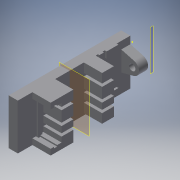
# Autodesk Inventor part: Assembly-jig-base
Saved by Autodesk Inventor 2018 (Build 220112000, 112)
## iProperties
Created: 2017-11-08
Part Number: Assembly-jig-base
Material: Generic
Document SubType Name: Modeling
Designer: xl0
Density: 1 g/cm^3
Appearance: Default
Author: xl0
Autodesk Inventor part; units mm, degrees
ref_plane "YZ Plane" through (0, 0, 0) normal (1, 0, 0) x (0, 1, 0)
ref_plane "XZ Plane" through (0, 0, 0) normal (0, 1, 0) x (-1, 0, 0)
ref_plane "XY Plane" through (0, 0, 0) normal (0, 0, 1) x (1, 0, 0)
ref_plane "Work Plane3" through (-2, 0, -40) normal (-1, 0, 0) x (0, 0, 1)
sketch "Sketch3" plane through (-2, 0, -8) normal (-1, 0, 0) x (0, -1, 0)
  line L0 (59.7526, 13.1) -> (72.7526, 13.1)
  line L1 (72.7526, 13.1) -> (72.7526, 3.1)
  line L2 (72.7526, 3.1) -> (59.7526, 3.1)
  line L3 (59.7526, 3.1) -> (59.7526, 13.1)
  line L4 (104.2526, 13.1) -> (117.2526, 13.1)
  line L5 (117.2526, 13.1) -> (117.2526, 3.1)
  line L6 (117.2526, 3.1) -> (104.2526, 3.1)
  line L7 (104.2526, 3.1) -> (104.2526, 13.1)
  line L8 (59.7526, -25.1) -> (72.7526, -25.1)
  line L9 (72.7526, -25.1) -> (72.7526, -35.1)
  line L10 (72.7526, -35.1) -> (59.7526, -35.1)
  line L11 (59.7526, -35.1) -> (59.7526, -25.1)
  line L12 (104.2526, -25.1) -> (117.2526, -25.1)
  line L13 (117.2526, -25.1) -> (117.2526, -35.1)
  line L14 (117.2526, -35.1) -> (104.2526, -35.1)
  line L15 (104.2526, -35.1) -> (104.2526, -25.1)
  line L16 (41.7526, -32) -> (41.7526, 8) projected
  line L17 (125.2526, 8) -> (125.2526, -32) projected
  line L18 (63.2526, 0) -> (63.2526, 3) projected
  line L19 (67.7526, 0) -> (67.7526, 3) projected
  line L20 (99.2526, 0) -> (99.2526, 3) projected
  line L21 (103.7526, 0) -> (103.7526, 3) projected
  line L22 (44.7526, 3) -> (122.2526, 3) projected
  line L23 (122.2526, -25) -> (44.7526, -25) projected
  line L24 (74.7526, -0.1) -> (87.7526, -0.1)
  line L25 (87.7526, -0.1) -> (87.7526, -11.9)
  line L26 (87.7526, -11.9) -> (74.7526, -11.9)
  line L27 (74.7526, -11.9) -> (74.7526, -0.1)
  line L28 (59.7526, -15.1) -> (72.7526, -15.1)
  line L29 (72.7526, -15.1) -> (72.7526, -21.9)
  line L30 (72.7526, -21.9) -> (59.7526, -21.9)
  line L31 (59.7526, -21.9) -> (59.7526, -15.1)
  line L32 (104.2526, -0.1) -> (117.2526, -0.1)
  line L33 (117.2526, -0.1) -> (117.2526, -11.9)
  line L34 (117.2526, -11.9) -> (104.2526, -11.9)
  line L35 (104.2526, -11.9) -> (104.2526, -0.1)
  line L36 (104.2526, -15.1) -> (117.2526, -15.1)
  line L37 (117.2526, -15.1) -> (117.2526, -21.9)
  line L38 (117.2526, -21.9) -> (104.2526, -21.9)
  line L39 (104.2526, -21.9) -> (104.2526, -15.1)
  line L40 (44.7526, 0) -> (122.2526, 0) projected
  line L41 (44.7526, -12) -> (122.2526, -12) projected
  line L42 (44.7526, -15) -> (122.2526, -15) projected
  line L43 (44.7526, -22) -> (122.2526, -22) projected
  line L44 (122.2526, 8) -> (122.2526, -32) projected
  line L45 (44.7526, -32) -> (44.7526, 8) projected
  line L46 (125.2526, 8) -> (122.2526, 8) projected
  line L47 (125.2526, -32) -> (122.2526, -32) projected
  dimension "d7" = 10
  dimension "d9" = 0.1
  dimension "d10" = 0.1
  dimension "d11" = 0.1
  dimension "d12" = 0.1
  dimension "d13" = 0.1
  dimension "d34" = 5
  dimension "d36" = 13
  dimension "d48" = 0.1
  dimension "d49" = 15
  dimension "d67" = 15
  constraints: 64 end point, 16 parallel, 14 collinear, 8 horizontal, 8 perpendicular, 4 equal length, 3 point on line
  measures "d7" distance of L0.end L1.end
  measures "d9" distance between parallel lines of L23 L8
  measures "d10" distance between parallel lines of L26 L41
  measures "d11" distance between parallel lines of L40 L24
  measures "d12" distance between parallel lines of L42 L28
  measures "d13" distance between parallel lines of L43 L30
  measures "d34" distance between parallel lines of L37 L44
  measures "d36" distance of L9.end L10.end
  measures "d48" distance between parallel lines of L22 L2
  measures "d49" distance between parallel lines of L45 L31
  measures "d67" distance between parallel lines of L27 L31
extrude "Extrusion2" add sketch "Sketch3" against normal blind 20 contours L0 L1 L2 L3 | L4 L5 L6 L7 | L8 L9 L10 L11 | L12 L13 L14 L15 | L24 L25 L26 L27 | L28 L29 L30 L31 | L32 L33 L34 L35 | L36 L37 L38 L39
sketch "Sketch10" plane through (-2, 0, -8) normal (-1, 0, 0) x (0, 0, 1)
  line L0 (13.1, -117.2526) -> (13.1, -129.2526)
  line L1 (13.1, -129.2526) -> (6.7, -129.2526)
  line L2 (6.7, -129.2526) -> (6.7, -125.4526)
  line L3 (6.7, -125.4526) -> (8.2, -125.4526)
  line L4 (6.7, -117.2526) -> (13.1, -117.2526)
  line L5 (8, -125.2526) -> (-32, -125.2526) projected
  line L6 (8, -125.2526) -> (8, -122.2526) projected
  line L7 (-32, -122.2526) -> (8, -122.2526) projected
  line L8 (-32, -125.2526) -> (-32, -122.2526) projected
  line L9 (13.1, -104.2526) -> (13.1, -117.2526) projected
  line L10 (-30.7, -129.2526) -> (-37.1, -129.2526)
  line L11 (-37.1, -129.2526) -> (-37.1, -104.2526)
  line L12 (-32.2, -125.4526) -> (-30.7, -125.4526)
  line L13 (-30.7, -125.4526) -> (-30.7, -129.2526)
  line L14 (-32.2, -125.4526) -> (-32.2, -122.0526)
  line L15 (-32.2, -122.0526) -> (-30.7, -122.0526)
  line L16 (-30.7, -122.0526) -> (-30.7, -117.2526)
  line L17 (8.2, -125.4526) -> (8.2, -122.0526)
  line L18 (8.2, -122.0526) -> (6.7, -122.0526)
  line L19 (6.7, -122.0526) -> (6.7, -117.2526)
  line L20 (13.1, -117.2526) -> (3.1, -117.2526) projected
  line L21 (-25.1, -104.2526) -> (-25.1, -117.2526) projected
  line L22 (-25.1, -117.2526) -> (-35.1, -117.2526) projected
  line L23 (-35.1, -117.2526) -> (-35.1, -104.2526) projected
  line L24 (-35.1, -104.2526) -> (-25.1, -104.2526) projected
  line L25 (-35.1, -117.2526) -> (-35.1, -104.2526) projected
  line L26 (-35.1, -104.2526) -> (-37.1, -104.2526)
  point P0 (8, 0)
  dimension "d50" = 0.2
  dimension "d54" = 12
  dimension "d58" = 0.2
  dimension "d59" = 0.2
  dimension "d60" = 1.5
  dimension "d61" = 0.2
  constraints: 32 end point, 9 collinear, 7 perpendicular, 3 horizontal, 3 parallel, 2 vertical, 1 point on line
  measures "d50" distance between parallel lines of L3 L5
  measures "d54" distance of L0.start L0.end
  measures "d58" distance between parallel lines of L17 L6
  measures "d59" distance between parallel lines of L18 L7
  measures "d60" distance of L17.end L18.end
  measures "d61" distance between parallel lines of L8 L14
extrude "Extrusion7" add sketch "Sketch10" against normal blind 20 contours L0 L1 L2 L3 L17 L18 L19 L4 | L10 L11 L26 L23 L22 L16 L15 L14 L12 L13
sketch "Sketch11" plane through (-2, 0, -8) normal (-1, 0, 0) x (0, 0, 1)
  line L0 (6.7, -122.0526) -> (6.7, -117.2526) projected
  line L1 (8.2, -122.0526) -> (6.7, -122.0526) projected
  line L2 (8.2, -125.4526) -> (8.2, -122.0526) projected
  line L3 (6.7, -125.4526) -> (8.2, -125.4526) projected
  line L4 (6.7, -129.2526) -> (6.7, -125.4526) projected
  line L5 (13.1, -129.2526) -> (6.7, -129.2526) projected
  line L6 (-37.1, -129.2526) -> (-30.7, -129.2526) projected
  line L7 (-30.7, -129.2526) -> (-30.7, -125.4526) projected
  line L8 (-30.7, -125.4526) -> (-32.2, -125.4526) projected
  line L9 (-32.2, -125.4526) -> (-32.2, -122.0526) projected
  line L10 (-32.2, -122.0526) -> (-30.7, -122.0526) projected
  line L11 (-30.7, -122.0526) -> (-30.7, -117.2526) projected
  line L12 (-37.1, -104.2526) -> (-37.1, -129.2526) projected
  line L13 (6.7, -122.0526) -> (6.7, -125.4526)
  line L14 (-30.7, -122.0526) -> (-32.2, -122.0526) projected
  line L15 (-30.7, -122.0526) -> (-30.7, -125.4526)
  line L16 (13.1, -36.7526) -> (6.1, -36.7526)
  line L17 (6.1, -36.7526) -> (6.1, -49.7526)
  line L18 (6.1, -49.7526) -> (13.1, -49.7526)
  line L19 (13.1, -49.7526) -> (13.1, -36.7526)
  line L20 (-28.1, -36.7526) -> (-35.1, -36.7526)
  line L21 (-35.1, -36.7526) -> (-35.1, -49.7526)
  line L22 (-35.1, -49.7526) -> (-28.1, -49.7526)
  line L23 (-28.1, -49.7526) -> (-28.1, -36.7526)
  line L24 (13.1, -59.7526) -> (13.1, -72.7526) projected
  line L25 (-35.1, -72.7526) -> (-35.1, -59.7526) projected
  line L26 (-11.9, -74.7526) -> (-0.1, -74.7526) projected
  line L27 (-32, -44.7526) -> (8, -44.7526)
  line L28 (-25.1, -104.2526) -> (-25.1, -117.2526) projected
  line L29 (-25.1, -117.2526) -> (-30.7, -117.2526) projected
  line L30 (13.1, -104.2526) -> (13.1, -129.2526) projected
  line L31 (3.1, -104.2526) -> (13.1, -104.2526) projected
  line L32 (3.1, -117.2526) -> (3.1, -104.2526) projected
  line L33 (6.7, -117.2526) -> (3.1, -117.2526) projected
  line L34 (-25.1, -104.2526) -> (-37.1, -104.2526) projected
  point P0 (8, 0)
  dimension "d64" = 7
  dimension "d65" = 5
  constraints: 22 end point, 5 collinear, 5 parallel, 3 horizontal, 3 perpendicular, 3 point on line, 2 other
  measures "d64" distance of L16.start L16.end
  measures "d65" distance between parallel lines of L22 L27
ref_plane "Work Plane5" through (0, -122.2526, -8) normal (-1, 0, 0) x (0, 0, 1)
extrude "Extrusion8" add sketch "Sketch11" against normal up to surface (2 mm away) contours L1 L2 L3 L13 | L12 L34 L28 L29 L11 L10 L9 L8 L7 L6 | L19 L18 L17 L16 | L23 L22 L21 L20
sketch "Sketch4" plane through (-2, 0, -8) normal (-1, 0, 0) x (0, 0, 1)
  line L0 (13.1, -21.7526) -> (-37.1, -21.7526)
  line L1 (-37.1, -21.7526) -> (-37.1, -130.2526)
  line L2 (-37.1, -130.2526) -> (13.1, -130.2526)
  line L3 (13.1, -130.2526) -> (13.1, -21.7526)
  line L4 (13.1, -59.7526) -> (13.1, -72.7526) projected
  line L5 (3.1, -59.7526) -> (13.1, -59.7526) projected
  line L6 (3.1, -72.7526) -> (3.1, -59.7526) projected
  line L7 (13.1, -72.7526) -> (3.1, -72.7526) projected
  line L8 (13.1, -104.2526) -> (13.1, -129.2526) projected
  line L9 (3.1, -104.2526) -> (13.1, -104.2526) projected
  line L10 (3.1, -117.2526) -> (3.1, -104.2526) projected
  line L11 (6.7, -117.2526) -> (3.1, -117.2526) projected
  line L12 (-25.1, -59.7526) -> (-25.1, -72.7526) projected
  line L13 (-35.1, -59.7526) -> (-25.1, -59.7526) projected
  line L14 (-35.1, -72.7526) -> (-35.1, -59.7526) projected
  line L15 (-25.1, -72.7526) -> (-35.1, -72.7526) projected
  line L16 (-25.1, -104.2526) -> (-25.1, -117.2526) projected
  line L17 (-25.1, -104.2526) -> (-37.1, -104.2526) projected
  line L18 (-25.1, -117.2526) -> (-30.7, -117.2526) projected
  line L19 (-32, -41.7526) -> (8, -41.7526) projected
  line L20 (8, -125.2526) -> (-32, -125.2526) projected
  line L21 (13.1, -59.7526) -> (13.1, -72.7526) projected
  line L22 (-35.1, -72.7526) -> (-35.1, -59.7526) projected
  line L23 (6.7, -129.2526) -> (6.7, -117.2526) projected
  line L24 (13.1, -129.2526) -> (6.7, -129.2526) projected
  line L25 (-37.1, -104.2526) -> (-37.1, -129.2526) projected
  line L26 (-37.1, -129.2526) -> (-30.7, -129.2526) projected
  line L27 (-30.7, -129.2526) -> (-30.7, -125.4526) projected
  line L28 (-30.7, -125.4526) -> (-32.2, -125.4526) projected
  line L29 (-32.2, -125.4526) -> (-32.2, -122.0526) projected
  line L30 (-32.2, -122.0526) -> (-30.7, -122.0526) projected
  line L31 (-30.7, -122.0526) -> (-30.7, -117.2526) projected
  line L32 (-37.1, -129.2526) -> (-37.1, -104.2526) projected
  point P0 (8, 0)
  dimension "d16" = 20
  dimension "d17" = 5
  constraints: 8 end point, 2 collinear, 2 parallel, 1 horizontal, 1 perpendicular
  measures "d16" distance between parallel lines of L0 L19
  measures "d17" distance between parallel lines of L2 L20
extrude "Extrusion3" add sketch "Sketch4" along normal blind 10 contours L3 L5 L6 L7 L9 L10 L11 L23 L24 L2 L1 L26 L27 L28 L29 L30 L31 L18 L16 L17 L0 | L3 L7 L6 L5 | L17 L16 L18 L31 L30 L29 L28 L27 L26 L1 | L3 L24 L23 L11 L10 L9 | L12 L15 L14 L13
sketch "Sketch5" plane through (-2, -21.7526, 5.1) normal (0, 1, 0) x (1, 0, 0)
  point P0 (2, 5.1)
sketch "Sketch6" plane through (-2, -21.7526, 5.1) normal (0, 1, 0) x (1, 0, 0)
  line L0 (26.75, 28.1) -> (18.75, 28.1) projected
  line L1 (18.75, 28.1) -> (18.75, 25.1) projected
  line L2 (26.75, 25.1) -> (18.75, 25.1) projected
  line L3 (26.75, 28.1) -> (26.75, 25.1) projected
  line L4 (26.75, 13.1) -> (18.75, 13.1) projected
  line L5 (18.75, 13.1) -> (18.75, 10.1) projected
  line L6 (26.75, 10.1) -> (18.75, 10.1) projected
  line L7 (26.75, 13.1) -> (26.75, 10.1) projected
  arc A0 (13.9411, 11.8556) -> (13.9411, 26.3444) centre (12, 19.1) ccw
  line L8 (20, 25) -> (20, 13.2) projected
  line L9 (0, 0) -> (0, 50.2) projected
  line L10 (13.9411, 26.3444) -> (0, 30.08)
  line L11 (0, 28.2) -> (0, 35) projected
  line L12 (13.9411, 11.8556) -> (0, 8.12)
  line L13 (0, 50.2) -> (0, 0) projected
  point P0 (2, 5.1)
  point P1 (20, 19.1)
  dimension "d20" = 8
  dimension "d21" = 15
  dimension "d22" = 75
  dimension "d23" = 75
  constraints: 4 end point, 2 point on circle, 2 point on line, 2 tangent, 1 centre point, 1 horizontal alignment, 1 midpoint
  measures "d20" distance from line of A0.centre L8
  measures "d21" diameter of A0
  measures "d22" angle of L13 L10
  measures "d23" angle of L9 L12
extrude "Extrusion4" add sketch "Sketch6" against normal blind 10 contours L12 L9 L10 A0
sketch "Sketch7" plane through (-2, -31.7526, 5.1) normal (0, -1, 0) x (1, 0, 0)
  arc A0 (13.9411, -26.3444) -> (13.9411, -11.8556) centre (12, -19.1) ccw projected
  line L0 (0, -8.12) -> (13.9411, -11.8556) projected
  line L1 (13.9411, -26.3444) -> (0, -30.08) projected
  point P0 (2, -5.1)
hole "Hole1" at (10, -31.7526, -14) direction (0, 1, 0) diameter 3 end through all counterbore diameter 7 counterbore depth 2
ref_plane "Work Plane4" through (18, -88.5026, -4.9) normal (0, -1, 0) x (1, 0, 0)
sketch "Sketch8" plane through (18, -72.7526, 5.1) normal (0, 0, 1) x (1, 0, 0)
  line L0 (-20, 51) -> (-20, 13) projected
  line L1 (-20, 20.5) -> (-18.5, 20.5)
  line L2 (-18.5, 20.5) -> (-18.5, 15.5)
  line L3 (-18.5, 15.5) -> (-20, 15.5)
  line L4 (-20, -15) -> (0, -15) projected
  line L5 (-20, 13) -> (0, 13) projected
  line L6 (-20, -15) -> (-9.8118, -15) construction
  line L7 (-20, 13) -> (-11.1239, 13) construction
  line L8 (-20, 13) -> (0, 13) construction
  line L9 (-20.9875, 18) -> (-11.746, 18) construction
  point P0 (-18, 72.7526)
  point P1 (-18, 13)
  dimension "d38" = 1.5
  dimension "d39" = 5
  dimension "d66" = 5
  constraints: 12 end point, 4 point on line, 3 perpendicular, 1 horizontal, 1 other
  measures "d38" distance between parallel lines of L0 L2
  measures "d39" distance between parallel lines of L3 L1
  measures "d66" distance between parallel lines of L9 L5
extrude "Extrusion5" add sketch "Sketch8" against normal up to surface (48.2 mm away)
mirror "Mirror1" about plane through (18, -88.5026, -4.9) normal (0, -1, 0) of "Extrusion5"
equation "\"d10\" = d9"
equation "\"d11\" = d9"
equation "\"d12\" = d9"
equation "\"d13\" = d9"
equation "\"d48\" = d9"
equation "\"d58\" = d50"
equation "\"d59\" = d50"
equation "\"d61\" = d50"
body "Solid2"
